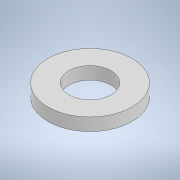
# Autodesk Inventor part: Bearing Washer
Saved by Autodesk Inventor 2022.2 (Build 262287000, 287)
## iProperties
Created: 2022-08-09
Part Number: Bearing Washer
Material: Generic
Document SubType Name: Modeling
Designer: Ilewicz
Density: 1 g/cm^3
Appearance: Default
Author: Ilewicz
Autodesk Inventor part; units mm, degrees
ref_plane "YZ Plane" through (0, 0, 0) normal (1, 0, 0) x (0, 1, 0)
ref_plane "XZ Plane" through (0, 0, 0) normal (0, 1, 0) x (-1, 0, 0)
ref_plane "XY Plane" through (0, 0, 0) normal (0, 0, 1) x (1, 0, 0)
sketch "Sketch1" plane through (0, 0, 0) normal (0, 1, 0) x (-1, 0, 0)
  circle A0 centre (0, 0) radius 2.5
  circle A1 centre (0, 0) radius 5
  dimension "d0" = 5
  dimension "d1" = 10
  constraints: 2 centre point, 2 coincident
  measures "d0" diameter of A0
  measures "d1" diameter of A1
extrude "Extrusion1" add sketch "Sketch1" along normal blind 1.5
body "Solid1"
